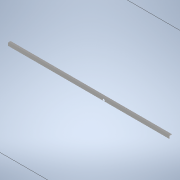
# Autodesk Inventor part: SP39V1 Chapa Acrilico
Saved by Autodesk Inventor 2021.2 (Build 252289000, 289)
## iProperties
Created: 2026-08-21
Part Number: SP39V1 Chapa Acrilico
Material: Generic
Document SubType Name: Sheet Metal
Designer: nelso
Density: 1 g/cm^3
Sheet Metal Rule: Default_mm
Appearance: Default
Author: nelso
Autodesk Inventor part; units mm, degrees
ref_plane "YZ Plane" through (0, 0, 0) normal (1, 0, 0) x (0, 1, 0)
ref_plane "XZ Plane" through (0, 0, 0) normal (0, 1, 0) x (-1, 0, 0)
ref_plane "XY Plane" through (0, 0, 0) normal (0, 0, 1) x (1, 0, 0)
sketch "Sketch1" plane through (0, 0, 0) normal (0, 1, 0) x (-1, 0, 0)
  line L0 (825, 15) -> (-825, 15)
  line L1 (-825, 15) -> (-825, -15)
  line L2 (-825, -15) -> (825, -15)
  line L3 (825, -15) -> (825, 15)
  line L4 (825, 15) -> (-825, -15) construction
  line L5 (-825, 15) -> (825, -15) construction
  point P0 (0, 0)
  dimension "d0" = 1650
  dimension "d1" = 30
  measures "d0" distance of L2.end L1.end
  measures "d1" distance of L1.end L0.end
extrude "Plate1" add sketch "Sketch1" along normal blind 3.2
sketch "Sketch2" plane through (825, 0, 11.8) normal (0, 0, 1) x (1, 0, 0)
  line L0 (-1650, 0) -> (0, 0)
  line L1 (0, 0) -> (0, 25)
  line L2 (0, 25) -> (-1650, 25)
  line L3 (-1650, 25) -> (-1650, 0)
  constraints: 6 end point, 1 horizontal, 1 perpendicular, 1 vertical
edge flange "Flange1" height 25 angle 90 thickness 3.2 bend radius 1.516 thickness toward (0, 0, 1) relief straight relief width 3.2 relief depth 1.6 edges at (0, 3.2, 15) wall of the first edge with corners at (-825, 0, 11.8) (825, 0, 11.8) (825, 25, 11.8) (-825, 25, 11.8)
bend "Bend1"
corner "Corner1"
sketch "Sketch3" plane through (825, 25, 11.8) normal (0, 0, -1) x (-1, 0, 0)
  circle A0 centre (105, -10.45) radius 1.5706 projected
  circle A1 centre (285, -10.45) radius 1.5706 projected
  circle A2 centre (465, -10.45) radius 1.5706 projected
  circle A3 centre (645, -10.45) radius 1.5706 projected
  circle A4 centre (825, -10.45) radius 1.5706 projected
  circle A5 centre (1005, -10.45) radius 1.5706 projected
  circle A6 centre (1185, -10.45) radius 1.5706 projected
  circle A7 centre (1365, -10.45) radius 1.5706 projected
  circle A8 centre (1545, -10.45) radius 1.5706 projected
  point P0 (825, -25)
hole "Hole1" at (540, 14.55, 11.8) at (720, 14.55, 11.8) at (360, 14.55, 11.8) at (180, 14.55, 11.8) at (0, 14.55, 11.8) at (-180, 14.55, 11.8) at (-360, 14.55, 11.8) at (-540, 14.55, 11.8) at (-720, 14.55, 11.8) direction (0, 0, 1) diameter 4.5 depth 3.2 tip angle 118 clearance for "Countersunk Flat Head Screw ISO 2009/7046" size "M4" standard "ISO"
sketch "Sketch4" plane through (0, 3.2, 0) normal (0, 1, 0) x (1, 0, 0)
  arc A0 (-825, 18.7) -> (-825, 25.3) centre (-825, 22) ccw projected
  line L0 (-825, 18.7) -> (-825, -14) projected
  line L1 (999.7, -14) -> (-825, -14) projected
  line L2 (999.7, 58) -> (999.7, -14) projected
  line L3 (-825, 58) -> (999.7, 58) projected
  line L4 (-825, 58) -> (-825, 25.3) projected
  circle A1 centre (161.541, 2) radius 10 projected
  circle A2 centre (946.4414, 33.8654) radius 11.11 projected
  line L5 (161.541, 2) -> (161.541, -25.5) construction
  line L6 (151.541, 2) -> (151.541, -25.5)
  line L7 (171.541, -25.5) -> (171.541, 2)
  arc A3 (171.541, 2) -> (151.541, 2) centre (161.541, 2) ccw
  arc A4 (151.541, -25.5) -> (171.541, -25.5) centre (161.541, -25.5) ccw
  line L8 (161.541, 2) -> (134.041, 2) construction
  line L9 (161.541, -8) -> (134.041, -8)
  line L10 (134.041, 12) -> (161.541, 12)
  arc A5 (161.541, -8) -> (161.541, 12) centre (161.541, 2) ccw
  arc A6 (134.041, 12) -> (134.041, -8) centre (134.041, 2) ccw
  line L11 (124.041, 2) -> (171.541, 2)
  line L12 (171.541, 2) -> (171.541, -14)
  line L13 (171.541, -14) -> (124.041, -14)
  line L14 (124.041, -14) -> (124.041, 2)
  point P0 (0, 0)
  point P1 (161.541, -11.75)
  point P2 (147.791, 2)
  dimension "d28" = 27.5
  dimension "d29" = 27.5
  constraints: 24 end point, 9 point on circle, 8 tangent, 4 centre point, 4 parallel, 2 concentric, 2 horizontal, 2 midpoint, 2 point on line, 1 perpendicular, 1 vertical
  measures "d28" distance of L5.start L5.end
  measures "d29" distance of L5.start L8.end
extrude "Cut1" cut sketch "Sketch4" against normal blind 3.2 contours L14 A6 L9 L6 L1 | L6 L9 A1 L7 L1 | L1 L7 A4 L6 | L11 L6 L9 A6 | A6 L10 A1 L11 | L6 A1 L9 | L11 A1 | A1 L11
sketch "Sketch7" plane through (-825, 25, 15) normal (0, 0, 1) x (1, 0, 0)
  line L0 (986.3019, -21.8) -> (986.3019, -25) projected
  line L1 (966.8022, -21.8) -> (986.3019, -21.8) projected
  line L2 (966.8022, -25) -> (966.8022, -21.8) projected
  line L3 (986.3019, -25) -> (966.8022, -25) projected
  line L4 (986.3019, -25) -> (946.3019, -25)
  line L5 (946.3019, -25) -> (946.3019, -21)
  line L6 (946.3019, -21) -> (986.3019, -21)
  line L7 (986.3019, -21) -> (986.3019, -25)
  point P0 (825, -25)
  dimension "d22" = 40
  dimension "d23" = 4
  constraints: 8 end point, 2 parallel, 1 horizontal, 1 perpendicular
  measures "d22" distance of L5.end L6.end
  measures "d23" distance of L4.end L5.end
extrude "Cut2" cut sketch "Sketch7" against normal blind 3.2 contours L1 L2 L4 L5 L6 L7
equation "\"d18\" = Thickness"
equation "\"d20\" = Thickness"
equation "\"d24\" = Thickness"
equation "\"d2\" = Thickness"
equation "\"d3\" = BendReliefWidth"
equation "\"d4\" = BendReliefDepth"
equation "\"d5\" = MinimumRemnant"
equation "\"d6\" = TransitionRadius"
equation "\"d9\" = BendRadius"
equation "\"d10\" = CornerReliefSize"
equation "\"d11\" = GapSize"
equation "\"d12\" = JacobiRadiusSize"
equation "\"BendReliefWidth\" = Thickness"
equation "\"BendReliefDepth\" = 0.5 * Thickness"
equation "\"CornerReliefSize\" = 4 * Thickness"
equation "\"MinimumRemnant\" = 2 * Thickness"
equation "\"TransitionRadius\" = BendRadius"
equation "\"JacobiRadiusSize\" = BendRadius"
equation "\"GapSize\" = Thickness"
equation "\"Thickness\" = 3.2"
equation "\"BendRadius\" = 1.516"
body "Solid1"
